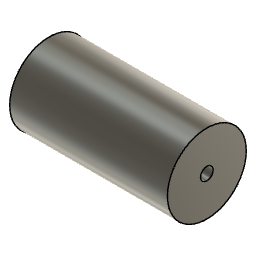
rueda suspension v2 (Autodesk Fusion 360 design; units mm, degrees)
Autodesk Fusion 360 part; units mm, degrees
sketch "Sketch1" plane through (0, 0, 0) normal (1, 0, 0) x (0, 1, 0)
  circle A0 centre (0, 0) radius 15
  line L0 (6.3897, -13.8986) -> (5.9544, -13.7676)
  line L1 (0, 15) -> (0, 23)
  line L2 (0, 15) -> (-3, 15)
  line L3 (0, 15) -> (3, 15)
  line L4 (0, 23) -> (3, 15)
  line L5 (0, 23) -> (-3, 15)
  line L6 (-3, 15) -> (-3.1925, 14.4866)
  line L7 (3, 15) -> (3.1794, 14.5216)
  circle A1 centre (0, 0) radius 15
  circle A2 centre (0, 0) radius 15
  line L8 (-23, 0) -> (-15, -3)
  line L9 (-23, 0) -> (-15, 3)
  line L10 (-15, 3) -> (-14.5216, 3.1794)
  line L11 (-15, -3) -> (-14.4866, -3.1925)
  circle A3 centre (0, 0) radius 15
  line L12 (0, -23) -> (3, -15)
  line L13 (0, -23) -> (-3, -15)
  line L14 (-3, -15) -> (-3.1794, -14.5216)
  line L15 (3, -15) -> (3.1925, -14.4866)
  circle A4 centre (0, 0) radius 15
  line L16 (23, 0) -> (15, 3)
  line L17 (23, 0) -> (15, -3)
  line L18 (15, -3) -> (14.5216, -3.1794)
  line L19 (15, 3) -> (14.4866, 3.1925)
  circle A5 centre (0, 0) radius 15
  dimension "d1" = 30
  dimension "d16" = 8
  dimension "d17" = 3
  dimension "d18" = 3
  dimension "d31" = 360
  constraint coincident A0.centre A1.centre
  constraint coincident A0 L1.start
  constraint vertical L1
  constraint perpendicular L1 L2
  constraint perpendicular L1 L3
  constraint parallel L5 L6
  constraint parallel L4 L7
  measures "d1" diameter of A0
  measures "d16" distance of L1.start L1.end
  measures "d17" distance of L1.start L2.end
  measures "d18" distance of L1.start L3.end
extrude "Extrude9" add sketch "Sketch1" along normal blind 60
sketch "Sketch8" plane through (60, 0, 0) normal (1, 0, 0) x (0, 1, 0)
  line L0 (23, 0) -> (14.6712, 3.1233)
  arc A0 (14.6712, 3.1233) -> (3.1233, 14.6712) centre (0, 0) ccw
  line L1 (3.1233, 14.6712) -> (0, 23)
  line L2 (0, 23) -> (-3.1233, 14.6712)
  arc A1 (-3.1233, 14.6712) -> (-14.6712, 3.1233) centre (0, 0) ccw
  line L3 (-14.6712, 3.1233) -> (-23, 0)
  line L4 (-23, 0) -> (-14.6712, -3.1233)
  arc A2 (-14.6712, -3.1233) -> (-3.1233, -14.6712) centre (0, 0) ccw
  line L5 (-3.1233, -14.6712) -> (0, -23)
  line L6 (0, -23) -> (3.1233, -14.6712)
  arc A3 (3.1233, -14.6712) -> (14.6712, -3.1233) centre (0, 0) ccw
  line L7 (14.6712, -3.1233) -> (23, 0)
  circle A4 centre (0, 0) radius 2.4
  dimension "d34" = 4.8
  constraint coincident A0.centre A1.centre
  measures "d34" diameter of A4
extrude "Extrude10" cut sketch "Sketch8" against normal blind 85 contours A4
sketch "Sketch9" plane through (60, 0, 0) normal (1, 0, 0) x (0, 1, 0)
  circle A0 centre (0, 0) radius 2.4
  line L0 (23, 0) -> (14.6712, 3.1233)
  arc A1 (14.6712, 3.1233) -> (3.1233, 14.6712) centre (0, 0) ccw
  line L1 (3.1233, 14.6712) -> (0, 23)
  line L2 (0, 23) -> (-3.1233, 14.6712)
  arc A2 (-3.1233, 14.6712) -> (-14.6712, 3.1233) centre (0, 0) ccw
  line L3 (-14.6712, 3.1233) -> (-23, 0)
  line L4 (-23, 0) -> (-14.6712, -3.1233)
  arc A3 (-14.6712, -3.1233) -> (-3.1233, -14.6712) centre (0, 0) ccw
  line L5 (-3.1233, -14.6712) -> (0, -23)
  line L6 (0, -23) -> (3.1233, -14.6712)
  arc A4 (3.1233, -14.6712) -> (14.6712, -3.1233) centre (0, 0) ccw
  line L7 (14.6712, -3.1233) -> (23, 0)
  circle A5 centre (0, 0) radius 23
  circle A6 centre (0, 0) radius 15
  constraint concentric A0 A5
  constraint coincident L0.start A5
  constraint concentric A5 A6
extrude "Extrude11" cut sketch "Sketch9" against normal blind 75 contours L0 L7 A6 | L1 L2 A6 | L5 L6 A6 | L3 L4 A6
sketch "Sketch10" plane through (0, 0, 0) normal (1, 0, 0) x (0, 1, 0)
  circle A0 centre (0, 0) radius 23
  circle A1 centre (0, 0) radius 15.0333
  constraint coincident A0.centre A1.centre
